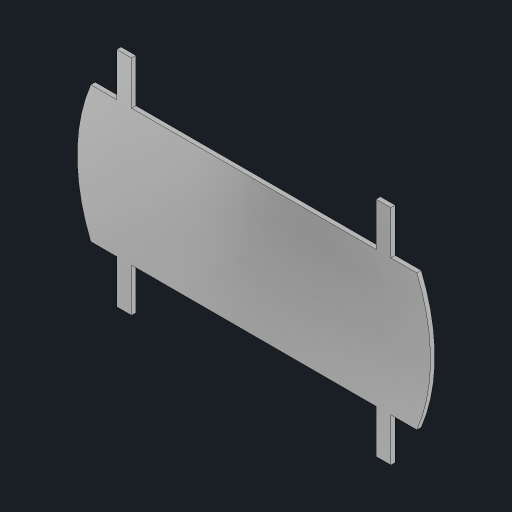
# Autodesk Inventor part: 1.6mm Aluminium Frame
Saved by Autodesk Inventor 2023.2 (Build 272271030, 271C)
## iProperties
Created: 2024-02-18
Part Number: 1.6mm Aluminium Frame
Material: Aluminum 6061
Document SubType Name: Modeling
Designer: robpl
Density: 2.7 g/cm^3
Appearance: Aluminum - Flat
Author: robpl
Autodesk Inventor part; units mm, degrees
ref_plane "YZ Plane" through (0, 0, 0) normal (1, 0, 0) x (0, 1, 0)
ref_plane "XZ Plane" through (0, 0, 0) normal (0, 1, 0) x (-1, 0, 0)
ref_plane "XY Plane" through (0, 0, 0) normal (0, 0, 1) x (1, 0, 0)
sketch "Sketch1" plane through (0, 0, 0) normal (0, 0, 1) x (1, 0, 0)
  circle A0 centre (0, 0) radius 65
  line L0 (60, -25) -> (-60, -25)
  line L1 (60, 25) -> (-60, 25)
  line L2 (45, -25) -> (50.4381, -25)
  line L3 (50.4381, -25) -> (50.4381, -41)
  line L4 (50.4381, -41) -> (45, -41)
  line L5 (45, -41) -> (45, -25)
  line L6 (-45, -25) -> (-50.4381, -25)
  line L7 (-50.4381, -25) -> (-50.4381, -41)
  line L8 (-50.4381, -41) -> (-45, -41)
  line L9 (-45, -41) -> (-45, -25)
  line L10 (45, 25) -> (50.4381, 25)
  line L11 (50.4381, 25) -> (50.4381, 41)
  line L12 (50.4381, 41) -> (45, 41)
  line L13 (45, 41) -> (45, 25)
  line L14 (-50.4381, 25) -> (-45, 25)
  line L15 (-45, 25) -> (-45, 41)
  line L16 (-45, 41) -> (-50.4381, 41)
  line L17 (-50.4381, 41) -> (-50.4381, 25)
  dimension "d0" = 130
  dimension "d1" = 50
  dimension "d2" = 90
  dimension "d4" = 16
  constraints: 36 end point, 8 parallel, 7 equal length, 6 horizontal, 4 perpendicular, 4 point on line, 1 coincident, 10 other
  measures "d1" distance between parallel lines of L0 L1
  measures "d2" distance between parallel lines of L13 L15
  measures "d4" distance of L12.end L10.start
extrude "Extrusion1" add sketch "Sketch1" along normal blind 1.6 contours A0 L0 L1 | L11 L1 L13 L12 | L4 L5 L0 L3 | L16 L15 L1 L17 | L7 L0 L9 L8
body "Solid1"
